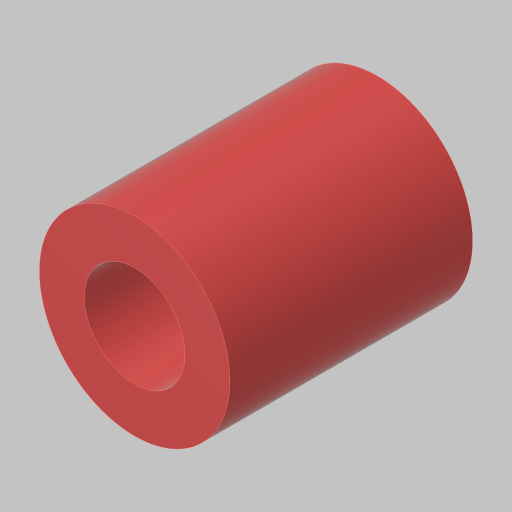
# Autodesk Inventor part: GP-SP-006
Saved by Autodesk Inventor 2023.5 (Build 275446000, 446)
## iProperties
Created: 2025-03-21
Part Number: GP-SP-006
Material: ABS Plastic
Document SubType Name: Modeling
Designer: slick
Density: 1.06 g/cm^3
Appearance: Smooth - Red
Author: slick
Autodesk Inventor part; units mm, degrees
ref_plane "YZ Plane" through (0, 0, 0) normal (1, 0, 0) x (0, 1, 0)
ref_plane "XZ Plane" through (0, 0, 0) normal (0, 1, 0) x (-1, 0, 0)
ref_plane "XY Plane" through (0, 0, 0) normal (0, 0, 1) x (1, 0, 0)
sketch "Sketch1" plane through (0, 0, 0) normal (0, 0, 1) x (1, 0, 0)
  circle A0 centre (0, 0) radius 7.112
  circle A1 centre (0, 0) radius 13.462
  dimension "d0" = 14.224
  dimension "d1" = 6.35
  constraints: 2 centre point, 1 coincident
  measures "d0" diameter of A0
  measures "d1" radial gap between concentric circles of A0 A1
extrude "Extrusion1" add sketch "Sketch1" along normal blind 34.29
body "Solid1"
